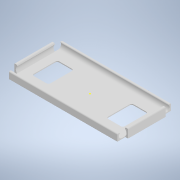
# Autodesk Inventor part: Part9
Saved by Autodesk Inventor 2020 (Build 240168000, 168)
## iProperties
Created: 2020-03-31
Part Number: Part9
Material: Generic
Document SubType Name: Modeling
Designer: Sverrir
Density: 1 g/cm^3
Appearance: Default
Author: Sverrir
Autodesk Inventor part; units mm, degrees
ref_plane "YZ Plane" through (0, 0, 0) normal (1, 0, 0) x (0, 1, 0)
ref_plane "XZ Plane" through (0, 0, 0) normal (0, 1, 0) x (-1, 0, 0)
ref_plane "XY Plane" through (0, 0, 0) normal (0, 0, 1) x (1, 0, 0)
sketch "Sketch1" plane through (0, 0, 0) normal (1, 0, 0) x (0, 1, 0)
  arc A0 (180, 810.64) -> (205, 835.64) centre (180, 835.64) ccw
  arc A1 (205, 858.7762) -> (173.7762, 890) centre (173.7762, 858.7762) ccw
  line L0 (0, 0) -> (30.28, 0) construction
  line L1 (205, 858.7762) -> (205, 835.64)
  line L2 (15, 0) -> (-15, 0) construction
  line L3 (-15, 0) -> (-15, 890)
  line L4 (15, 0) -> (15, 737.14)
  line L5 (0, 0) -> (0, 51.3695) construction
  line L6 (173.7762, 890) -> (-15, 890)
  line L7 (119.6029, 0) -> (249.4149, 0) construction
  spline S0 degree 4 poles (15, 737.14) (15, 762.8587) (22.661, 806.5882) (93.3132, 851.1722) (153.9624, 839.5046) (176.9487, 823.6651) (180, 810.64) knots 0 0 0 0 0 0.365063 0.584044 1 1 1 1 1
  line L8 (238.5148, 856.7698) -> (95.5367, 856.7698) construction
  line L9 (93.5, 837.14) -> (143.5, 837.14) construction
  line L10 (118.5, 837.14) -> (118.5, 840) construction
  line L11 (180, -810.64) -> (180, -810.64)
  arc A2 (205, -835.64) -> (180, -810.64) centre (180, -835.64) ccw
  arc A3 (173.7762, -890) -> (205, -858.7762) centre (173.7762, -858.7762) ccw
  line L12 (205, -858.7762) -> (205, -835.64)
  line L13 (-15, 0) -> (-15, -890)
  line L14 (15, 0) -> (15, -737.14)
  line L15 (173.7762, -890) -> (-15, -890)
  spline S1 degree 4 poles (15, -737.14) (15, -762.8587) (22.661, -806.5882) (93.3132, -851.1722) (153.9624, -839.5046) (176.9487, -823.6651) (180, -810.64) knots 0 0 0 0 0 0.365063 0.584044 1 1 1 1 1
  line L16 (180, 810.64) -> (162.5735, 810.64) construction
  point P0 (178.1248, 805.5246)
  point P1 (35.5, 803.14)
  point P2 (170.5, 824.64)
  point P3 (35.5, -803.14)
  point P4 (93.5, -837.14)
  point P5 (143.5, -837.14)
  point P6 (170.5, -824.64)
  point P7 (180, -810.64)
  dimension "d145" = 23.1363
  dimension "d151" = 30
  dimension "d161" = 165
  dimension "d324" = 9.5
  dimension "d325" = 27
  dimension "d326" = 50
  dimension "d327" = 58
  dimension "d328" = 66
  dimension "d329" = 34
  dimension "d330" = 14
  dimension "d331" = 12.5
  dimension "d332" = 840
  dimension "d333" = 50
  dimension "d349" = 90
  dimension "d350" = 220
  constraints: 36 end point, 13 symmetric about line, 9 point on circle, 7 horizontal, 6 vertical, 4 centre point, 3 tangent, 2 midpoint, 1 point on line, 17 other
  measures "d145" distance of L1.start L1.end
  measures "d151" distance between parallel lines of L3 L4
  measures "d161" distance from line of L4 L16.start
  measures "d324" horizontal distance of L16.start point (170.5, 824.64)
  measures "d325" horizontal distance of point (170.5, 824.64) L9.end
  measures "d326" distance of L9.end L9.start
  measures "d327" horizontal distance of L9.start point (35.5, 803.14)
  measures "d328" vertical distance of point (35.5, 803.14) L4.end
  measures "d329" vertical distance of point (35.5, 803.14) L9.start
  measures "d330" vertical distance of point (170.5, 824.64) L16.start
  measures "d331" vertical distance of point (170.5, 824.64) L9.end
  measures "d332" vertical distance of L0.start L10.end
  measures "d333" distance from line of L6 L10.end
  measures "d350" distance between parallel lines of L1 L3
sketch "Sketch2" plane through (0, 0, 0) normal (0, 0, 1) x (1, 0, 0)
  line L0 (-1794.8732, 15) -> (-1828.3732, 45) construction
  spline S0 degree 4 poles (-1794.8732, 15) (-1828.3732, 45) (-1847.3732, 115) (-1834.3732, 151) (-1810.3732, 196) (-1786.4748, 223) knots 1 1 1 1 1 1.747458 2 2 2 2 2
  line L1 (-1810.3732, 196) -> (-1786.4748, 223) construction
  line L2 (-1828.3732, 45) -> (-1847.3732, 115) construction
  line L3 (-1847.3732, 115) -> (-1834.3732, 151) construction
  line L4 (-1834.3732, 151) -> (-1810.3732, 196) construction
  line L5 (-1835.9285, 190.8381) -> (-1835.9285, 47.3152) construction
  line L6 (-1885.9285, -15) -> (-1885.9285, 237.5463)
  line L7 (0, 0) -> (20, 0) construction
  line L8 (0, 0) -> (0, 15) construction
  line L9 (0, 15) -> (-1794.8732, 15)
  line L10 (-1858.4748, 265) -> (-1828.4748, 265)
  arc A0 (-1858.4748, 265) -> (-1885.9285, 237.5463) centre (-1858.4748, 237.5463) ccw
  arc A1 (-1786.4748, 223) -> (-1828.4748, 265) centre (-1828.4748, 223) ccw
  line L11 (-1835.9285, -15) -> (0, -15)
  line L12 (-1885.9285, -15) -> (-1835.9285, -15)
  line L13 (1786.4748, 223) -> (1786.4748, 223)
  spline S1 degree 4 poles (1794.8732, 15) (1828.3732, 45) (1847.3732, 115) (1834.3732, 151) (1810.3732, 196) (1786.4748, 223) knots 1 1 1 1 1 1.747458 2 2 2 2 2
  line L14 (1794.8732, 15) -> (1828.3732, 45) construction
  line L15 (1828.3732, 45) -> (1847.3732, 115) construction
  line L16 (1847.3732, 115) -> (1834.3732, 151) construction
  line L17 (1834.3732, 151) -> (1810.3732, 196) construction
  line L18 (1810.3732, 196) -> (1786.4748, 223) construction
  line L19 (1885.9285, -15) -> (1885.9285, 237.5463)
  line L20 (0, 15) -> (1794.8732, 15)
  line L21 (1858.4748, 265) -> (1828.4748, 265)
  arc A2 (1885.9285, 237.5463) -> (1858.4748, 265) centre (1858.4748, 237.5463) ccw
  arc A3 (1828.4748, 265) -> (1786.4748, 223) centre (1828.4748, 223) ccw
  line L22 (1835.9285, -15) -> (0, -15)
  line L23 (1885.9285, -15) -> (1835.9285, -15)
  line L24 (-1836.4162, 120.7995) -> (1835.4407, 120.7995) construction
  line L25 (1835.4407, 215.7869) -> (1835.4407, 25.812) construction
  line L26 (1835.4407, 25.812) -> (-1836.4162, 25.812) construction
  line L27 (-1836.4162, 25.812) -> (-1836.4162, 215.7869) construction
  line L28 (-1836.4162, 215.7869) -> (1835.4407, 215.7869) construction
  line L29 (1835.9285, 207.1179) -> (1835.9285, 57.9131) construction
  point P0 (1786.4748, 223)
  point P1 (-1835.9285, 119.0766)
  dimension "d132" = 27
  dimension "d133" = 45
  dimension "d134" = 36
  dimension "d135" = 70
  dimension "d136" = 30
  dimension "d137" = 33.5
  dimension "d138" = 19
  dimension "d139" = 13
  dimension "d140" = 24
  dimension "d141" = 23.8984
  dimension "d169" = 30
  dimension "d174" = 250
  dimension "d176" = 1835.9285
  dimension "d177" = 30
  dimension "d178" = 50
  dimension "d179" = 20
  dimension "d336" = 90
  dimension "d345" = 3671.8569
  constraints: 33 end point, 14 symmetric about line, 8 point on circle, 6 horizontal, 6 vertical, 4 centre point, 3 midpoint, 3 tangent, 2 point on line, 12 other
  measures "d132" vertical distance of L1.end L4.end
  measures "d133" vertical distance of L3.end L4.end
  measures "d134" vertical distance of L3.end L2.end
  measures "d135" vertical distance of L2.end L0.end
  measures "d136" vertical distance of L0.end L0.start
  measures "d137" horizontal distance of L0.end L0.start
  measures "d138" horizontal distance of L0.end L2.end
  measures "d139" horizontal distance of L3.end L2.end
  measures "d140" horizontal distance of L3.end L4.end
  measures "d141" horizontal distance of L4.end L1.end
  measures "d169" distance of L10.start L10.end
  measures "d174" distance between parallel lines of L9 L10
  measures "d176" distance of L11.start L11.end
  measures "d177" distance between parallel lines of L11 L9
  measures "d178" distance from line of L5 L6.end
  measures "d179" distance of L7.start L7.end
  measures "d345" distance between parallel lines of L29 L5
extrude "Extrusion3" add sketch "Sketch1" against normal mid plane 3600
extrude "Extrusion4" add sketch "Sketch2" along normal mid plane 1250
sketch "Sketch4" plane through (-1789.2984, 15, 559.8188) normal (0, 1, 0) x (1, 0, 0)
  line L0 (3676.7725, 1250) -> (3676.7725, 0) projected
  line L1 (3296.7725, 979.8188) -> (2746.7725, 979.8188)
  line L2 (2746.7725, 979.8188) -> (2746.7725, 139.8188)
  line L3 (2746.7725, 139.8188) -> (3296.7725, 139.8188)
  line L4 (3296.7725, 139.8188) -> (3296.7725, 979.8188)
  line L5 (4431.453, 559.8188) -> (-851.3105, 559.8188) projected
  line L6 (1789.2984, 1805.8188) -> (1789.2984, -686.1812) projected
  line L7 (831.8244, 979.8188) -> (281.8244, 979.8188)
  line L8 (281.8244, 979.8188) -> (281.8244, 139.8188)
  line L9 (281.8244, 139.8188) -> (831.8244, 139.8188)
  line L10 (831.8244, 139.8188) -> (831.8244, 979.8188)
  point P0 (1789.2984, 559.8188)
  dimension "d90" = 420
  dimension "d91" = 420
  dimension "d92" = 550
  dimension "d93" = 380
  dimension "d98" = 957.474
  dimension "d99" = 957.474
  dimension "d100" = 550
  constraints: 16 end point, 4 parallel, 2 collinear, 2 horizontal, 2 perpendicular
  measures "d90" distance between parallel lines of L5 L1
  measures "d91" distance between parallel lines of L5 L3
  measures "d92" distance between parallel lines of L2 L4
  measures "d93" distance between parallel lines of L0 L4
  measures "d98" distance between parallel lines of L2 L6
  measures "d99" distance between parallel lines of L6 L10
  measures "d100" distance between parallel lines of L10 L8
extrude "Extrusion5" cut sketch "Sketch4" against normal blind 1200
fillet "Fillet1" radius 63.5 8 edges at (1507.474, 0, 420) (957.474, 0, 420) (957.474, 0, -420) (1507.474, 0, -420) (-1507.474, 0, -420) (-957.474, 0, -420) (-1507.474, 0, 420) (-957.474, 0, 420)
sketch "Sketch11" plane through (-1800, 15, -725.6356) normal (0, 1, 0) x (1, 0, 0)
  point P0 (1800, -725.6356)
body "Solid2"
